Autodesk Fusion 360 part; units mm, degrees
note: some values were not read from the file. Chosen so that the rebuilt part matches the saved one: which face or edge a step refers to; which pieces of a blend or face edit are solid. Set by a fixed rule: which sketch regions a step uses.
(part 2 of 5)
  line L115 (-88.0068, -37.0951) -> (-84.7252, -33.8135)
  arc A155 (49.1749, 62.2927) -> (41.7643, 61.9168) centre (45.6394, 58.7571) ccw
  line L116 (38.5865, -65.8101) -> (15.8059, -43.0296)
  line L117 (-65.8101, -38.5865) -> (-43.0296, -15.8059)
  line L118 (-42.4797, -62.6322) -> (-23.3401, -43.4926)
  arc A156 (84.7263, -33.8146) -> (84.7252, -33.8135) centre (81.1896, -37.349) ccw
  line L119 (0, 0) -> (0, -10)
  arc A157 (84.7252, -33.8135) -> (77.6541, -33.8135) centre (81.1896, -37.349) ccw
  line L120 (33.8327, -77.6349) -> (33.8316, -77.636)
  line L121 (38.6227, -72.8449) -> (33.8139, -77.6537)
  arc A158 (-49.1749, -62.2927) -> (-41.7643, -61.9168) centre (-45.6394, -58.7571) ccw
  line L122 (77.653, -33.8146) -> (77.6541, -33.8135)
  line L123 (72.8449, -38.6227) -> (72.863, -38.6046)
  line L124 (-84.7081, -33.8327) -> (-84.707, -33.8316)
  line L125 (-38.6046, -72.863) -> (-72.8811, -38.5865)
  arc A159 (38.5865, -72.8811) -> (38.5865, -65.8101) centre (35.0509, -69.3456) ccw
  arc A160 (-72.8811, -38.5865) -> (-65.8101, -38.5865) centre (-69.3456, -35.0509) ccw
  line L126 (42.122, -62.2745) -> (23.3401, -43.4926)
  arc A161 (62.2745, 42.122) -> (62.2745, 49.1931) centre (58.739, 45.6575) ccw
  line L127 (62.6322, -42.4797) -> (43.4926, -23.3401)
  line L128 (-42.122, 62.2745) -> (-23.3401, 43.4926)
  arc A162 (-65.4524, 38.2288) -> (-72.863, 38.6046) centre (-69.3275, 35.0691) ccw
  line L129 (62.2745, 42.122) -> (43.4926, 23.3401)
  line L130 (-72.863, 38.6046) -> (-77.6541, 33.8135)
  arc A163 (65.4524, -38.2288) -> (72.863, -38.6046) centre (69.3275, -35.0691) ccw
  arc A164 (33.8139, -77.6537) -> (33.7586, -84.6686) centre (37.3495, -81.1892) ccw
  line L131 (-55.7429, 55.7247) -> (-52.8534, 52.8352)
  arc A165 (-62.2745, -42.122) -> (-62.2745, -49.1931) centre (-58.739, -45.6575) ccw
  line L132 (-38.5865, 65.8101) -> (-15.8059, 43.0296)
  arc A166 (-38.5865, 72.8811) -> (-38.5865, 65.8101) centre (-35.0509, 69.3456) ccw
  line L133 (66.1678, -38.9441) -> (43.0296, -15.8059)
  line L134 (72.8449, 38.6227) -> (77.636, 33.8316)
  line L135 (72.8449, -38.6227) -> (77.6541, -33.8135)
  line L136 (38.6227, -72.8449) -> (38.5865, -72.8811)
  line L137 (42.4797, 62.6322) -> (23.3401, 43.4926)
  line L138 (35.2277, -86.1394) -> (33.8135, -84.7252)
  line L139 (87.9887, 37.1133) -> (84.707, 33.8316)
  line L140 (-37.1133, 87.9887) -> (-33.8316, 84.707)
  arc A167 (42.122, -62.2745) -> (49.1931, -62.2745) centre (45.6575, -58.739) ccw
  line L141 (37.0951, 88.0068) -> (33.8135, 84.7252)
  line L142 (-62.2745, -42.122) -> (-43.4926, -23.3401)
  line L143 (-77.636, -33.8316) -> (-77.6541, -33.8135)
  arc A168 (-33.8327, 77.6349) -> (-33.8327, 84.7081) centre (-37.3672, 81.1715) ccw
  arc A169 (62.2927, -49.1749) -> (61.9168, -41.7643) centre (58.7571, -45.6394) ccw
  line L144 (38.6046, 72.863) -> (33.8135, 77.6541)
  line L145 (-38.6046, -72.863) -> (-33.8135, -77.6541)
  line L146 (33.8135, -84.7252) -> (33.7586, -84.6686)
  line L147 (72.863, -38.6046) -> (38.5865, -72.8811)
  line L148 (-66.1678, 38.9441) -> (-43.0296, 15.8059)
  arc A170 (-33.8146, -84.7263) -> (-33.8146, -77.653) centre (-37.349, -81.1896) ccw
  line L149 (-72.8449, -38.6227) -> (-77.636, -33.8316)
  line L150 (-37.0951, -88.0068) -> (-33.8135, -84.7252)
  arc A171 (-77.6541, -33.8135) -> (-84.7252, -33.8135) centre (-81.1896, -37.349) ccw
  point P0 (-86.1394, -35.2277)
  point P1 (35.2277, -86.1394)
  point P2 (86.1394, 35.2277)
  point P3 (86.1394, 35.2277)
  point P4 (-86.1394, -35.2277)
  point P5 (35.2277, -86.1394)
  dimension "d63" = 5
  dimension "d64" = 5
  dimension "d67" = 5
  dimension "d82" = 5
  dimension "d83" = 5
  dimension "d84" = 5
  constraint concentric A25 A123
  constraint concentric A76 A124
  constraint concentric A77 A125
  constraint concentric A81 A126
  constraint coincident A25.start L16.start
  constraint coincident L16.end A26.end
  constraint coincident L39.end A76.end
  constraint coincident L39.start A80.start
  constraint coincident A77.start L41.start
  constraint tangent L64 A125
  constraint parallel L41 L64
  constraint coincident A81.end L45.end
  constraint coincident A88.start L45.start
  constraint coincident L15.end A25.end
  constraint coincident A24.end L15.start
  constraint coincident A23.start L14.start
  constraint coincident L14.end A24.start
  constraint concentric A24 A122
  constraint coincident A24.end A122
  constraint coincident L14 A122.start
  constraint coincident L15 A122.end
  constraint coincident L16 A123.start
  constraint coincident L39 A124.end
  constraint midpoint L40 L68.start
  constraint perpendicular L40 L68
  constraint symmetric L15.end L68 L70.start
  constraint symmetric A24.end L68 L70.end
  constraint symmetric A23.start L68 L69.start
  constraint symmetric L14.end L68 L69.end
  constraint symmetric A122 L68 A127
  constraint symmetric A122.start L68 A127.end
  constraint symmetric A122.end L68 A127.start
  constraint coincident L13.end A21.end
  constraint tangent A21 L95
  constraint perpendicular L95 L96
  constraint tangent L96 A144
  constraint tangent L95 A144
  constraint coincident A5.centre A10.centre
  constraint vertical L97
  constraint symmetric L74.start L97 L98.start
  constraint coincident A63.start L29.start
  constraint tangent A63 L99
  constraint perpendicular L99 L100
  constraint tangent L99 A145
  constraint tangent L100 A145
  constraint collinear L101 L102
  constraint parallel L81 L103
  constraint coincident P5 P1
  constraint perpendicular L103 L104
  constraint parallel L3 L105
  constraint tangent L103 A146
  constraint tangent L105 A146
  constraint tangent A152 L128
  constraint coincident A24.end A151
  constraint symmetric L15.end L70.start L131
  constraint symmetric A24.end L70.end L131
  constraint symmetric A23.start L69.start L131
  constraint symmetric L14.end L69.end L131
  constraint symmetric A151 L131 A168
  constraint symmetric A122.start A127.end L131
  constraint symmetric A122.end A127.start L131
  constraint perpendicular L115 L143
  constraint tangent L143 A171
  constraint tangent L115 A171
  constraint vertical L119
  constraint symmetric L74.start L98.start L119
  constraint perpendicular L107 L135
  constraint tangent L107 A157
  constraint tangent A157 L135
  constraint collinear L120 L136
  constraint parallel L121 L147
  constraint perpendicular L121 L138
  constraint tangent L121 A164
  constraint tangent A164 L146
  measures "d63" radius of A144
  measures "d64" radius of A145
  measures "d67" radius of A146
  measures "d82" radius of A171
  measures "d83" radius of A157
  measures "d84" radius of A164
extrude "押し出し10" cut sketch "スケッチ2" against normal blind 100 contours L6 A12 L7 A13 A128 L72 A132 A148 L145 A170 | A14 L9 A15 L73 L77 A130 A131 A158 L125 A165 L142 | A19 L12 A20 L13 L73 L74 A129 L76 L96 A144 L117 L125 A160 L143 L149 A171 | A7 L2 A8 L3 L81 A134 L101 L103 A146 L121 A159 A164 L136 L147 | L36 L81 A135 A136 A167 A169 L147 | L29 A64 L30 A65 A133 L81 A137 L84 L98 L100 A145 A156 A157 L123 A163 L133 L135 L147 | A118 L53 L54 A119 L55 L56 A120 L57 L58 A121 L59 L60 bodies 1
extrude "押し出し11" add sketch "スケッチ2" against normal blind 1.5 contours L36 L37 L38 A135 A167 | L35 L36 A136 A169 bodies 1
sketch "スケッチ4" plane through (0, 0, 0) normal (0, 0, -1) x (1, 0, 0)
  arc A0 (17.125, 34.0956) -> (-17.125, 34.0956) centre (0, 0) ccw
  line L0 (17.125, 34.0956) -> (17.1965, 34.167)
  line L1 (17.1965, 34.167) -> (17.4152, 33.9483)
  arc A1 (33.9483, 17.4152) -> (17.4152, 33.9483) centre (0, 0) ccw
  line L2 (33.9483, 17.4152) -> (34.167, 17.1965)
  line L3 (34.167, 17.1965) -> (34.0956, 17.125)
  arc A2 (-34.0956, 17.125) -> (34.0956, 17.125) centre (0, 0) ccw
  line L4 (-34.0956, 17.125) -> (-34.167, 17.1965)
  line L5 (-34.167, 17.1965) -> (-33.9483, 17.4152)
  arc A3 (-17.4152, 33.9483) -> (-33.9483, 17.4152) centre (0, 0) ccw
  line L6 (-17.4152, 33.9483) -> (-17.1965, 34.167)
  line L7 (-17.1965, 34.167) -> (-17.125, 34.0956)
  circle A4 centre (-39.2089, -15.5208) radius 1.75
  circle A5 centre (-15.5208, -39.2089) radius 1.75
  circle A6 centre (-26.1275, -49.8155) radius 1.75
  circle A7 centre (-49.8155, -26.1275) radius 1.75
  arc A8 (32.3993, 86.1394) -> (35.2277, 86.1394) centre (33.8135, 87.5536) ccw
  line L8 (32.3993, 86.1394) -> (26.1835, 92.3551)
  arc A9 (25.9652, 94.9247) -> (26.1835, 92.3551) centre (27.5978, 93.7693) ccw
  arc A10 (25.9652, 94.9247) -> (26.3162, 95.431) centre (0, 113.3) ccw
  arc A11 (32.0144, 97.3721) -> (26.3162, 95.431) centre (30.4528, 92.6222) ccw
  arc A12 (39.6929, 94.5025) -> (32.0144, 97.3721) centre (0, 0) ccw
  arc A13 (40.3326, 91.2443) -> (39.6929, 94.5025) centre (38.9184, 92.6585) ccw
  line L9 (40.3326, 91.2443) -> (35.2277, 86.1394)
  circle A14 centre (26.1275, 49.8155) radius 1.75
  arc A15 (23.3401, 43.4926) -> (24.0851, 35.8083) centre (26.8756, 39.9571) ccw
  line L10 (23.3401, 43.4926) -> (42.122, 62.2745)
  arc A16 (49.1931, 62.2745) -> (42.122, 62.2745) centre (45.6575, 58.739) ccw
  line L11 (49.1931, 62.2745) -> (62.2927, 49.1749)
  arc A17 (62.6322, 42.4797) -> (62.2927, 49.1749) centre (58.7571, 45.6394) ccw
  line L12 (62.6322, 42.4797) -> (43.4926, 23.3401)
  arc A18 (35.8083, 24.0851) -> (43.4926, 23.3401) centre (39.9571, 26.8756) ccw
  arc A19 (35.8083, 24.0851) -> (24.0851, 35.8083) centre (0, 0) ccw
  circle A20 centre (49.8155, -26.1275) radius 1.75
  circle A21 centre (49.8155, 26.1275) radius 1.75
  circle A22 centre (15.5208, 39.2089) radius 1.75
  circle A23 centre (26.1275, -49.8155) radius 1.75
  circle A24 centre (39.2089, 15.5208) radius 1.75
  circle A25 centre (15.5208, -39.2089) radius 1.75
  circle A26 centre (39.2089, -15.5208) radius 1.75
  line L13 (-35.2277, 86.1394) -> (-40.3326, 91.2443)
  arc A27 (-39.6929, 94.5025) -> (-40.3326, 91.2443) centre (-38.9184, 92.6585) ccw
  arc A28 (-32.0144, 97.3721) -> (-39.6929, 94.5025) centre (0, 0) ccw
  arc A29 (-26.3162, 95.431) -> (-32.0144, 97.3721) centre (-30.4528, 92.6222) ccw
  arc A30 (-26.3162, 95.431) -> (-25.9652, 94.9247) centre (0, 113.3) ccw
  arc A31 (-26.1835, 92.3551) -> (-25.9652, 94.9247) centre (-27.5978, 93.7693) ccw
  line L14 (-26.1835, 92.3551) -> (-32.3993, 86.1394)
  arc A32 (-35.2277, 86.1394) -> (-32.3993, 86.1394) centre (-33.8135, 87.5536) ccw
  arc A33 (-38.5865, 72.8811) -> (-38.5865, 65.8101) centre (-35.0509, 69.3456) ccw
  line L15 (-38.5865, 72.8811) -> (-24.7285, 86.7391)
  arc A34 (-18.3143, 87.2917) -> (-24.7285, 86.7391) centre (-21.193, 83.2035) ccw
  arc A35 (-18.3143, 87.2917) -> (18.3143, 87.2917) centre (0, 113.3) ccw
  arc A36 (24.7285, 86.7391) -> (18.3143, 87.2917) centre (21.193, 83.2035) ccw
  line L16 (24.7285, 86.7391) -> (38.5865, 72.8811)
  arc A37 (38.5865, 65.8101) -> (38.5865, 72.8811) centre (35.0509, 69.3456) ccw
  line L17 (38.5865, 65.8101) -> (15.8059, 43.0296)
  arc A38 (10.9963, 41.7301) -> (15.8059, 43.0296) centre (12.2704, 46.5651) ccw
  arc A39 (10.9963, 41.7301) -> (-10.9963, 41.7301) centre (0, 0) ccw
  arc A40 (-15.8059, 43.0296) -> (-10.9963, 41.7301) centre (-12.2704, 46.5651) ccw
  line L18 (-15.8059, 43.0296) -> (-38.5865, 65.8101)
  line L19 (-43.4926, 23.3401) -> (-62.6322, 42.4797)
  arc A41 (-62.2927, 49.1749) -> (-62.6322, 42.4797) centre (-58.7571, 45.6394) ccw
  line L20 (-62.2927, 49.1749) -> (-49.1931, 62.2745)
  arc A42 (-42.122, 62.2745) -> (-49.1931, 62.2745) centre (-45.6575, 58.739) ccw
  line L21 (-42.122, 62.2745) -> (-23.3401, 43.4926)
  arc A43 (-24.0851, 35.8083) -> (-23.3401, 43.4926) centre (-26.8756, 39.9571) ccw
  arc A44 (-24.0851, 35.8083) -> (-35.8083, 24.0851) centre (0, 0) ccw
  arc A45 (-43.4926, 23.3401) -> (-35.8083, 24.0851) centre (-39.9571, 26.8756) ccw
  arc A46 (62.2927, -49.1749) -> (62.6322, -42.4797) centre (58.7571, -45.6394) ccw
  line L22 (62.2927, -49.1749) -> (49.1931, -62.2745)
  arc A47 (42.122, -62.2745) -> (49.1931, -62.2745) centre (45.6575, -58.739) ccw
  line L23 (42.122, -62.2745) -> (23.3401, -43.4926)
  arc A48 (24.0851, -35.8083) -> (23.3401, -43.4926) centre (26.8756, -39.9571) ccw
  arc A49 (24.0851, -35.8083) -> (35.8083, -24.0851) centre (0, 0) ccw
  arc A50 (43.4926, -23.3401) -> (35.8083, -24.0851) centre (39.9571, -26.8756) ccw
  line L24 (43.4926, -23.3401) -> (62.6322, -42.4797)
  arc A51 (84.7252, -33.8135) -> (77.6541, -33.8135) centre (81.1896, -37.349) ccw
  line L25 (77.6541, -33.8135) -> (72.863, -38.6046)
  arc A52 (66.1678, -38.9441) -> (72.863, -38.6046) centre (69.3275, -35.0691) ccw
  line L26 (66.1678, -38.9441) -> (63.9577, -36.7341)
  line L27 (63.9577, -36.7341) -> (43.0296, -15.8059)
  arc A53 (41.7301, -10.9963) -> (43.0296, -15.8059) centre (46.5651, -12.2704) ccw
  arc A54 (41.7301, -10.9963) -> (41.7301, 10.9963) centre (0, 0) ccw
  arc A55 (43.0296, 15.8059) -> (41.7301, 10.9963) centre (46.5651, 12.2704) ccw
  line L28 (43.0296, 15.8059) -> (66.1678, 38.9441)
  arc A56 (72.863, 38.6046) -> (66.1678, 38.9441) centre (69.3275, 35.0691) ccw
  line L29 (72.863, 38.6046) -> (77.6541, 33.8135)
  arc A57 (77.6541, 33.8135) -> (84.7252, 33.8135) centre (81.1896, 37.349) ccw
  line L30 (84.7252, 33.8135) -> (88.0068, 37.0951)
  arc A58 (96.2368, 35.2806) -> (88.0068, 37.0951) centre (91.5424, 33.5596) ccw
  arc A59 (96.2368, -35.2806) -> (96.2368, 35.2806) centre (0, 0) ccw
  arc A60 (88.0068, -37.0951) -> (96.2368, -35.2806) centre (91.5424, -33.5596) ccw
  line L31 (88.0068, -37.0951) -> (84.7252, -33.8135)
  arc A61 (-90.783, -46.7156) -> (-91.4938, -47.061) centre (-91.0045, -47.1639) ccw
  arc A62 (-90.783, -46.7156) -> (-89.7814, -45.9408) centre (-93.3169, -42.4052) ccw
  line L32 (-89.7814, -45.9408) -> (-84.7252, -40.8846)
  arc A63 (-77.6541, -40.8846) -> (-84.7252, -40.8846) centre (-81.1896, -44.4201) ccw
  line L33 (-77.6541, -40.8846) -> (-40.8846, -77.6541)
  arc A64 (-40.8846, -84.7252) -> (-40.8846, -77.6541) centre (-44.4201, -81.1896) ccw
  line L34 (-40.8846, -84.7252) -> (-45.9408, -89.7814)
  arc A65 (-45.9408, -89.7814) -> (-44.4738, -97.869) centre (-42.4052, -93.3169) ccw
  arc A66 (-44.4738, -97.869) -> (44.4738, -97.869) centre (0, 0) ccw
  arc A67 (44.4738, -97.869) -> (45.9408, -89.7814) centre (42.4052, -93.3169) ccw
  line L35 (45.9408, -89.7814) -> (40.8846, -84.7252)
  arc A68 (40.8846, -77.6541) -> (40.8846, -84.7252) centre (44.4201, -81.1896) ccw
  line L36 (40.8846, -77.6541) -> (77.6541, -40.8846)
  arc A69 (84.7252, -40.8846) -> (77.6541, -40.8846) centre (81.1896, -44.4201) ccw
  line L37 (84.7252, -40.8846) -> (89.7814, -45.9408)
  arc A70 (89.7814, -45.9408) -> (90.783, -46.7156) centre (93.3169, -42.4052) ccw
  arc A71 (91.4938, -47.061) -> (90.783, -46.7156) centre (91.0045, -47.1639) ccw
  arc A72 (91.4938, -47.061) -> (97.869, -44.4738) centre (93.3169, -42.4052) ccw
  arc A73 (97.869, -44.4738) -> (97.869, 44.4738) centre (0, 0) ccw
  arc A74 (97.869, 44.4738) -> (89.7814, 45.9408) centre (93.3169, 42.4052) ccw
  line L38 (89.7814, 45.9408) -> (84.7252, 40.8846)
  arc A75 (77.6541, 40.8846) -> (84.7252, 40.8846) centre (81.1896, 44.4201) ccw
  line L39 (77.6541, 40.8846) -> (40.8846, 77.6541)
  arc A76 (40.8846, 84.7252) -> (40.8846, 77.6541) centre (44.4201, 81.1896) ccw
  line L40 (40.8846, 84.7252) -> (45.9408, 89.7814)
  arc A77 (45.9408, 89.7814) -> (44.4738, 97.869) centre (42.4052, 93.3169) ccw
  arc A78 (44.4738, 97.869) -> (37.9262, 100.5876) centre (0, 0) ccw
  arc A79 (37.9256, 100.5859) -> (37.9262, 100.5876) centre (0, 113.3) ccw
  arc A80 (37.9256, 100.5859) -> (37.8014, 100.6345) centre (36.0432, 95.9538) ccw
  arc A81 (37.8014, 100.6345) -> (29.5575, 103.3567) centre (0, 0) ccw
  arc A82 (29.5575, 103.3567) -> (23.7528, 100.868) centre (28.1827, 98.5494) ccw
  arc A83 (-23.7528, 100.868) -> (23.7528, 100.868) centre (0, 113.3) ccw
  arc A84 (-23.7528, 100.868) -> (-29.5575, 103.3567) centre (-28.1827, 98.5494) ccw
  arc A85 (-29.5575, 103.3567) -> (-37.8014, 100.6345) centre (0, 0) ccw
  arc A86 (-37.8014, 100.6345) -> (-37.9256, 100.5859) centre (-36.0432, 95.9538) ccw
  arc A87 (-37.9262, 100.5876) -> (-37.9256, 100.5859) centre (0, 113.3) ccw
  arc A88 (-37.9262, 100.5876) -> (-44.4738, 97.869) centre (0, 0) ccw
  arc A89 (-44.4738, 97.869) -> (-45.9408, 89.7814) centre (-42.4052, 93.3169) ccw
  line L41 (-45.9408, 89.7814) -> (-40.8846, 84.7252)
  arc A90 (-40.8846, 77.6541) -> (-40.8846, 84.7252) centre (-44.4201, 81.1896) ccw
  line L42 (-40.8846, 77.6541) -> (-77.6541, 40.8846)
  arc A91 (-84.7252, 40.8846) -> (-77.6541, 40.8846) centre (-81.1896, 44.4201) ccw
  line L43 (-84.7252, 40.8846) -> (-89.7814, 45.9408)
  arc A92 (-89.7814, 45.9408) -> (-97.869, 44.4738) centre (-93.3169, 42.4052) ccw
  arc A93 (-97.869, 44.4738) -> (-97.869, -44.4738) centre (0, 0) ccw
  arc A94 (-97.869, -44.4738) -> (-91.4938, -47.061) centre (-93.3169, -42.4052) ccw
  line L44 (-63.9577, -36.7341) -> (-65.8101, -38.5865)
  arc A95 (-72.8811, -38.5865) -> (-65.8101, -38.5865) centre (-69.3456, -35.0509) ccw
  line L45 (-72.8811, -38.5865) -> (-77.6541, -33.8135)
  arc A96 (-77.6541, -33.8135) -> (-84.7252, -33.8135) centre (-81.1896, -37.349) ccw
  line L46 (-84.7252, -33.8135) -> (-88.0068, -37.0951)
  arc A97 (-96.2368, -35.2806) -> (-88.0068, -37.0951) centre (-91.5424, -33.5596) ccw
  arc A98 (-96.2368, 35.2806) -> (-96.2368, -35.2806) centre (0, 0) ccw
  arc A99 (-88.0068, 37.0951) -> (-96.2368, 35.2806) centre (-91.5424, 33.5596) ccw
  line L47 (-88.0068, 37.0951) -> (-84.7252, 33.8135)
  arc A100 (-84.7252, 33.8135) -> (-77.6541, 33.8135) centre (-81.1896, 37.349) ccw
  line L48 (-77.6541, 33.8135) -> (-72.863, 38.6046)
  arc A101 (-66.1678, 38.9441) -> (-72.863, 38.6046) centre (-69.3275, 35.0691) ccw
  line L49 (-66.1678, 38.9441) -> (-43.0296, 15.8059)
  arc A102 (-41.7301, 10.9963) -> (-43.0296, 15.8059) centre (-46.5651, 12.2704) ccw
  arc A103 (-41.7301, 10.9963) -> (-41.7301, -10.9963) centre (0, 0) ccw
  arc A104 (-43.0296, -15.8059) -> (-41.7301, -10.9963) centre (-46.5651, -12.2704) ccw
  line L50 (-43.0296, -15.8059) -> (-63.9577, -36.7341)
  arc A105 (-49.1749, -62.2927) -> (-42.4797, -62.6322) centre (-45.6394, -58.7571) ccw
  line L51 (-49.1749, -62.2927) -> (-62.2745, -49.1931)
  arc A106 (-62.2745, -42.122) -> (-62.2745, -49.1931) centre (-58.739, -45.6575) ccw
  line L52 (-62.2745, -42.122) -> (-43.4926, -23.3401)
  arc A107 (-35.8083, -24.0851) -> (-43.4926, -23.3401) centre (-39.9571, -26.8756) ccw
  arc A108 (-35.8083, -24.0851) -> (-24.0851, -35.8083) centre (0, 0) ccw
  arc A109 (-23.3401, -43.4926) -> (-24.0851, -35.8083) centre (-26.8756, -39.9571) ccw
  line L53 (-23.3401, -43.4926) -> (-42.4797, -62.6322)
  arc A110 (-33.7038, -84.612) -> (-33.8146, -77.653) centre (-37.349, -81.1896) ccw
  line L54 (-33.8146, -77.653) -> (-38.6046, -72.863)
  arc A111 (-38.9441, -66.1678) -> (-38.6046, -72.863) centre (-35.0691, -69.3275) ccw
  line L55 (-38.9441, -66.1678) -> (-15.8059, -43.0296)
  arc A112 (-10.9963, -41.7301) -> (-15.8059, -43.0296) centre (-12.2704, -46.5651) ccw
  arc A113 (-10.9963, -41.7301) -> (10.9963, -41.7301) centre (0, 0) ccw
  arc A114 (15.8059, -43.0296) -> (10.9963, -41.7301) centre (12.2704, -46.5651) ccw
  line L56 (15.8059, -43.0296) -> (38.9441, -66.1678)
  arc A115 (38.9491, -66.2144) -> (38.9441, -66.1678) centre (33.9744, -66.7173) ccw
  arc A116 (38.5865, -72.8811) -> (38.9491, -66.2144) centre (35.0509, -69.3456) ccw
  line L57 (38.5865, -72.8811) -> (33.8139, -77.6537)
  arc A117 (33.8139, -77.6537) -> (33.7586, -84.6686) centre (37.3495, -81.1892) ccw
  line L58 (33.7586, -84.6686) -> (33.8135, -84.7252)
  line L59 (33.8135, -84.7252) -> (37.0951, -88.0068)
  arc A118 (35.2806, -96.2368) -> (37.0951, -88.0068) centre (33.5596, -91.5424) ccw
  arc A119 (-35.2806, -96.2368) -> (35.2806, -96.2368) centre (0, 0) ccw
  arc A120 (-37.0951, -88.0068) -> (-35.2806, -96.2368) centre (-33.5596, -91.5424) ccw
  line L60 (-37.0951, -88.0068) -> (-33.8135, -84.7252)
  line L61 (-33.8135, -84.7252) -> (-33.7038, -84.612)
  circle A121 centre (-49.8155, 26.1275) radius 1.75
  circle A122 centre (-15.5208, 39.2089) radius 1.75
  circle A123 centre (-39.2089, 15.5208) radius 1.75
  circle A124 centre (-26.1275, 49.8155) radius 1.75
  circle A125 centre (-32.1379, -59.3615) radius 1.75
  circle A126 centre (32.1379, -59.3615) radius 1.75
  circle A127 centre (-32.1379, -59.3615) radius 2.5
  circle A128 centre (32.1379, -59.3615) radius 2.5
  dimension "d89" = 3.5
  dimension "d90" = 3.5
  dimension "d91" = 5
  dimension "d92" = 5
  constraint concentric A125 A127
  constraint concentric A126 A128
  measures "d89" diameter of A125
  measures "d90" diameter of A126
  measures "d91" diameter of A127
  measures "d92" diameter of A128
extrude "押し出し12" add sketch "スケッチ4" against normal blind 1.5 contours L55 A125 A127 | L55 A125 A127 | L56 A126 A128 picked at (33.5684, -61.0906) bodies 1
extrude "押し出し13" cut sketch "スケッチ4" against normal blind 1.5 contours L55 A125 | L55 A125 | L56 A126 picked at (32.0241, -58.7893) bodies 1
fillet "フィレット4" radius 5 4 edges at (-30.3701, 57.5937, 0.75) (-33.9056, 61.1292, 0.75) (33.9056, 61.1292, 0.75) (30.3701, 57.5937, 0.75) on bodies 1
sketch "スケッチ5" plane through (0, 0, 1.5) normal (0, 0, 1) x (-1, 0, 0)
  circle A0 centre (39.2089, -15.5208) radius 1.75
  circle A1 centre (15.5208, -39.2089) radius 1.75
  circle A2 centre (26.1275, -49.8155) radius 1.75
  circle A3 centre (49.8155, -26.1275) radius 1.75
  arc A4 (-35.2277, 86.1394) -> (-32.3993, 86.1394) centre (-33.8135, 87.5536) ccw
  line L0 (-35.2277, 86.1394) -> (-40.3326, 91.2443)
  arc A5 (-39.6929, 94.5025) -> (-40.3326, 91.2443) centre (-38.9184, 92.6585) ccw
  arc A6 (-32.0144, 97.3721) -> (-39.6929, 94.5025) centre (0, 0) ccw
  arc A7 (-26.3162, 95.431) -> (-32.0144, 97.3721) centre (-30.4528, 92.6222) ccw
  arc A8 (-26.3162, 95.431) -> (-25.9652, 94.9247) centre (0, 113.3) ccw
  arc A9 (-26.1835, 92.3551) -> (-25.9652, 94.9247) centre (-27.5978, 93.7693) ccw
  line L1 (-26.1835, 92.3551) -> (-32.3993, 86.1394)
  circle A10 centre (-26.1275, 49.8155) radius 1.75
  arc A11 (-24.0851, 35.8083) -> (-23.3401, 43.4926) centre (-26.8756, 39.9571) ccw
  arc A12 (-24.0851, 35.8083) -> (-35.8083, 24.0851) centre (0, 0) ccw
  arc A13 (-43.4926, 23.3401) -> (-35.8083, 24.0851) centre (-39.9571, 26.8756) ccw
  line L2 (-43.4926, 23.3401) -> (-62.6322, 42.4797)
  arc A14 (-62.2927, 49.1749) -> (-62.6322, 42.4797) centre (-58.7571, 45.6394) ccw
  line L3 (-62.2927, 49.1749) -> (-49.1931, 62.2745)
  arc A15 (-42.122, 62.2745) -> (-49.1931, 62.2745) centre (-45.6575, 58.739) ccw
  line L4 (-42.122, 62.2745) -> (-23.3401, 43.4926)
  circle A16 centre (-49.8155, -26.1275) radius 1.75
  circle A17 centre (-49.8155, 26.1275) radius 1.75
  circle A18 centre (-15.5208, 39.2089) radius 1.75
  circle A19 centre (-26.1275, -49.8155) radius 1.75
  circle A20 centre (-39.2089, 15.5208) radius 1.75
  circle A21 centre (-15.5208, -39.2089) radius 1.75
  circle A22 centre (-39.2089, -15.5208) radius 1.75
  line L5 (40.3326, 91.2443) -> (35.2277, 86.1394)
  arc A23 (32.3993, 86.1394) -> (35.2277, 86.1394) centre (33.8135, 87.5536) ccw
  line L6 (32.3993, 86.1394) -> (26.1835, 92.3551)
  arc A24 (25.9652, 94.9247) -> (26.1835, 92.3551) centre (27.5978, 93.7693) ccw
  arc A25 (25.9652, 94.9247) -> (26.3162, 95.431) centre (0, 113.3) ccw
  arc A26 (32.0144, 97.3721) -> (26.3162, 95.431) centre (30.4528, 92.6222) ccw
  arc A27 (39.6929, 94.5025) -> (32.0144, 97.3721) centre (0, 0) ccw
  arc A28 (40.3326, 91.2443) -> (39.6929, 94.5025) centre (38.9184, 92.6585) ccw
  arc A29 (17.125, 34.0956) -> (-17.125, 34.0956) centre (0, 0) ccw
  line L7 (17.125, 34.0956) -> (17.1965, 34.167)
  line L8 (17.1965, 34.167) -> (17.4152, 33.9483)
  arc A30 (33.9483, 17.4152) -> (17.4152, 33.9483) centre (0, 0) ccw
  line L9 (33.9483, 17.4152) -> (34.167, 17.1965)
  line L10 (34.167, 17.1965) -> (34.0956, 17.125)
  arc A31 (-34.0956, 17.125) -> (34.0956, 17.125) centre (0, 0) ccw
  line L11 (-34.0956, 17.125) -> (-34.167, 17.1965)
  line L12 (-34.167, 17.1965) -> (-33.9483, 17.4152)
  arc A32 (-17.4152, 33.9483) -> (-33.9483, 17.4152) centre (0, 0) ccw
  line L13 (-17.4152, 33.9483) -> (-17.1965, 34.167)
  line L14 (-17.1965, 34.167) -> (-17.125, 34.0956)
  line L15 (38.5865, 65.8101) -> (15.8059, 43.0296)
  arc A33 (10.9963, 41.7301) -> (15.8059, 43.0296) centre (12.2704, 46.5651) ccw
  arc A34 (10.9963, 41.7301) -> (-10.9963, 41.7301) centre (0, 0) ccw
  arc A35 (-15.8059, 43.0296) -> (-10.9963, 41.7301) centre (-12.2704, 46.5651) ccw
  line L16 (-15.8059, 43.0296) -> (-38.5865, 65.8101)
  arc A36 (-38.5865, 72.8811) -> (-38.5865, 65.8101) centre (-35.0509, 69.3456) ccw
  line L17 (-38.5865, 72.8811) -> (-24.7285, 86.7391)
  arc A37 (-18.3143, 87.2917) -> (-24.7285, 86.7391) centre (-21.193, 83.2035) ccw
  arc A38 (-18.3143, 87.2917) -> (18.3143, 87.2917) centre (0, 113.3) ccw
  arc A39 (24.7285, 86.7391) -> (18.3143, 87.2917) centre (21.193, 83.2035) ccw
  line L18 (24.7285, 86.7391) -> (38.5865, 72.8811)
  arc A40 (38.5865, 65.8101) -> (38.5865, 72.8811) centre (35.0509, 69.3456) ccw
  line L19 (62.6322, 42.4797) -> (43.4926, 23.3401)
  arc A41 (35.8083, 24.0851) -> (43.4926, 23.3401) centre (39.9571, 26.8756) ccw
  arc A42 (35.8083, 24.0851) -> (24.0851, 35.8083) centre (0, 0) ccw
  arc A43 (23.3401, 43.4926) -> (24.0851, 35.8083) centre (26.8756, 39.9571) ccw
  line L20 (23.3401, 43.4926) -> (42.122, 62.2745)
  arc A44 (49.1931, 62.2745) -> (42.122, 62.2745) centre (45.6575, 58.739) ccw
  line L21 (49.1931, 62.2745) -> (62.2927, 49.1749)
  arc A45 (62.6322, 42.4797) -> (62.2927, 49.1749) centre (58.7571, 45.6394) ccw
  arc A46 (91.4938, -47.061) -> (90.783, -46.7156) centre (91.0045, -47.1639) ccw
  arc A47 (91.4938, -47.061) -> (97.869, -44.4738) centre (93.3169, -42.4052) ccw
  arc A48 (97.869, -44.4738) -> (97.869, 44.4738) centre (0, 0) ccw
  arc A49 (97.869, 44.4738) -> (89.7814, 45.9408) centre (93.3169, 42.4052) ccw
  line L22 (89.7814, 45.9408) -> (84.7252, 40.8846)
  arc A50 (77.6541, 40.8846) -> (84.7252, 40.8846) centre (81.1896, 44.4201) ccw
  line L23 (77.6541, 40.8846) -> (40.8846, 77.6541)
  arc A51 (40.8846, 84.7252) -> (40.8846, 77.6541) centre (44.4201, 81.1896) ccw
  line L24 (40.8846, 84.7252) -> (45.9408, 89.7814)
  arc A52 (45.9408, 89.7814) -> (44.4738, 97.869) centre (42.4052, 93.3169) ccw
  arc A53 (44.4738, 97.869) -> (37.9262, 100.5876) centre (0, 0) ccw
  arc A54 (37.9256, 100.5859) -> (37.9262, 100.5876) centre (0, 113.3) ccw
  arc A55 (37.9256, 100.5859) -> (37.8014, 100.6345) centre (36.0432, 95.9538) ccw
  arc A56 (37.8014, 100.6345) -> (29.5575, 103.3567) centre (0, 0) ccw
  arc A57 (29.5575, 103.3567) -> (23.7528, 100.868) centre (28.1827, 98.5494) ccw
  arc A58 (-23.7528, 100.868) -> (23.7528, 100.868) centre (0, 113.3) ccw
  arc A59 (-23.7528, 100.868) -> (-29.5575, 103.3567) centre (-28.1827, 98.5494) ccw
  arc A60 (-29.5575, 103.3567) -> (-37.8014, 100.6345) centre (0, 0) ccw
  arc A61 (-37.8014, 100.6345) -> (-37.9256, 100.5859) centre (-36.0432, 95.9538) ccw
  arc A62 (-37.9262, 100.5876) -> (-37.9256, 100.5859) centre (0, 113.3) ccw
  arc A63 (-37.9262, 100.5876) -> (-44.4738, 97.869) centre (0, 0) ccw
  arc A64 (-44.4738, 97.869) -> (-45.9408, 89.7814) centre (-42.4052, 93.3169) ccw
  line L25 (-45.9408, 89.7814) -> (-40.8846, 84.7252)
  arc A65 (-40.8846, 77.6541) -> (-40.8846, 84.7252) centre (-44.4201, 81.1896) ccw
  line L26 (-40.8846, 77.6541) -> (-77.6541, 40.8846)
  arc A66 (-84.7252, 40.8846) -> (-77.6541, 40.8846) centre (-81.1896, 44.4201) ccw
  line L27 (-84.7252, 40.8846) -> (-89.7814, 45.9408)
  arc A67 (-89.7814, 45.9408) -> (-97.869, 44.4738) centre (-93.3169, 42.4052) ccw
  arc A68 (-97.869, 44.4738) -> (-97.869, -44.4738) centre (0, 0) ccw
  arc A69 (-97.869, -44.4738) -> (-91.4938, -47.061) centre (-93.3169, -42.4052) ccw
  arc A70 (-90.783, -46.7156) -> (-91.4938, -47.061) centre (-91.0045, -47.1639) ccw
  arc A71 (-90.783, -46.7156) -> (-89.7814, -45.9408) centre (-93.3169, -42.4052) ccw
  line L28 (-89.7814, -45.9408) -> (-84.7252, -40.8846)
  arc A72 (-77.6541, -40.8846) -> (-84.7252, -40.8846) centre (-81.1896, -44.4201) ccw
  line L29 (-77.6541, -40.8846) -> (-40.8846, -77.6541)
  arc A73 (-40.8846, -84.7252) -> (-40.8846, -77.6541) centre (-44.4201, -81.1896) ccw
  line L30 (-40.8846, -84.7252) -> (-45.9408, -89.7814)
  arc A74 (-45.9408, -89.7814) -> (-44.4738, -97.869) centre (-42.4052, -93.3169) ccw
  arc A75 (-44.4738, -97.869) -> (44.4738, -97.869) centre (0, 0) ccw
  arc A76 (44.4738, -97.869) -> (45.9408, -89.7814) centre (42.4052, -93.3169) ccw
  line L31 (45.9408, -89.7814) -> (40.8846, -84.7252)
  arc A77 (40.8846, -77.6541) -> (40.8846, -84.7252) centre (44.4201, -81.1896) ccw
  line L32 (40.8846, -77.6541) -> (77.6541, -40.8846)
  arc A78 (84.7252, -40.8846) -> (77.6541, -40.8846) centre (81.1896, -44.4201) ccw
  line L33 (84.7252, -40.8846) -> (89.7814, -45.9408)
  arc A79 (89.7814, -45.9408) -> (90.783, -46.7156) centre (93.3169, -42.4052) ccw
  circle A80 centre (49.8155, 26.1275) radius 1.75
  circle A81 centre (15.5208, 39.2089) radius 1.75
  circle A82 centre (39.2089, 15.5208) radius 1.75
  circle A83 centre (26.1275, 49.8155) radius 1.75
  line L34 (65.8101, -38.5865) -> (63.9577, -36.7341)
  line L35 (63.9577, -36.7341) -> (43.0296, -15.8059)
  arc A84 (41.7301, -10.9963) -> (43.0296, -15.8059) centre (46.5651, -12.2704) ccw
  arc A85 (41.7301, -10.9963) -> (41.7301, 10.9963) centre (0, 0) ccw
  arc A86 (43.0296, 15.8059) -> (41.7301, 10.9963) centre (46.5651, 12.2704) ccw
  line L36 (43.0296, 15.8059) -> (66.1678, 38.9441)
  arc A87 (72.863, 38.6046) -> (66.1678, 38.9441) centre (69.3275, 35.0691) ccw
  line L37 (72.863, 38.6046) -> (77.6541, 33.8135)
  arc A88 (77.6541, 33.8135) -> (84.7252, 33.8135) centre (81.1896, 37.349) ccw
  line L38 (84.7252, 33.8135) -> (88.0068, 37.0951)
  arc A89 (96.2368, 35.2806) -> (88.0068, 37.0951) centre (91.5424, 33.5596) ccw
  arc A90 (96.2368, -35.2806) -> (96.2368, 35.2806) centre (0, 0) ccw
  arc A91 (88.0068, -37.0951) -> (96.2368, -35.2806) centre (91.5424, -33.5596) ccw
  line L39 (88.0068, -37.0951) -> (84.7252, -33.8135)
  arc A92 (84.7252, -33.8135) -> (77.6541, -33.8135) centre (81.1896, -37.349) ccw
  line L40 (77.6541, -33.8135) -> (72.8811, -38.5865)
  arc A93 (65.8101, -38.5865) -> (72.8811, -38.5865) centre (69.3456, -35.0509) ccw
  arc A94 (42.4797, -62.6322) -> (49.1749, -62.2927) centre (45.6394, -58.7571) ccw
  line L41 (42.4797, -62.6322) -> (23.3401, -43.4926)
  arc A95 (24.0851, -35.8083) -> (23.3401, -43.4926) centre (26.8756, -39.9571) ccw
  arc A96 (24.0851, -35.8083) -> (35.8083, -24.0851) centre (0, 0) ccw
  arc A97 (43.4926, -23.3401) -> (35.8083, -24.0851) centre (39.9571, -26.8756) ccw
  line L42 (43.4926, -23.3401) -> (62.2745, -42.122)
  arc A98 (62.2745, -49.1931) -> (62.2745, -42.122) centre (58.739, -45.6575) ccw
  line L43 (62.2745, -49.1931) -> (49.1749, -62.2927)
  arc A99 (-77.6541, -33.8135) -> (-84.7252, -33.8135) centre (-81.1896, -37.349) ccw
  line L44 (-84.7252, -33.8135) -> (-88.0068, -37.0951)
  arc A100 (-96.2368, -35.2806) -> (-88.0068, -37.0951) centre (-91.5424, -33.5596) ccw
  arc A101 (-96.2368, 35.2806) -> (-96.2368, -35.2806) centre (0, 0) ccw
  arc A102 (-88.0068, 37.0951) -> (-96.2368, 35.2806) centre (-91.5424, 33.5596) ccw
  line L45 (-88.0068, 37.0951) -> (-84.7252, 33.8135)
  arc A103 (-84.7252, 33.8135) -> (-77.6541, 33.8135) centre (-81.1896, 37.349) ccw
  line L46 (-77.6541, 33.8135) -> (-72.863, 38.6046)
  arc A104 (-66.1678, 38.9441) -> (-72.863, 38.6046) centre (-69.3275, 35.0691) ccw
  line L47 (-66.1678, 38.9441) -> (-43.0296, 15.8059)
  arc A105 (-41.7301, 10.9963) -> (-43.0296, 15.8059) centre (-46.5651, 12.2704) ccw
  arc A106 (-41.7301, 10.9963) -> (-41.7301, -10.9963) centre (0, 0) ccw
  arc A107 (-43.0296, -15.8059) -> (-41.7301, -10.9963) centre (-46.5651, -12.2704) ccw
  line L48 (-43.0296, -15.8059) -> (-63.9577, -36.7341)
  line L49 (-63.9577, -36.7341) -> (-66.1678, -38.9441)
  arc A108 (-72.863, -38.6046) -> (-66.1678, -38.9441) centre (-69.3275, -35.0691) ccw
  line L50 (-72.863, -38.6046) -> (-77.6541, -33.8135)
  arc A109 (29.6417, -59.2224) -> (32.277, -61.8576) centre (32.1379, -59.3615) ccw
  arc A110 (36.0907, -63.3143) -> (32.277, -61.8576) centre (32.5552, -66.8499) ccw
  line L51 (36.0907, -63.3143) -> (38.9441, -66.1678)
  arc A111 (38.6046, -72.863) -> (38.9441, -66.1678) centre (35.0691, -69.3275) ccw
  line L52 (38.6046, -72.863) -> (33.8146, -77.653)
  arc A112 (33.8146, -77.653) -> (33.7038, -84.612) centre (37.349, -81.1896) ccw
  line L53 (33.7038, -84.612) -> (33.8135, -84.7252)
  line L54 (33.8135, -84.7252) -> (37.0951, -88.0068)
  arc A113 (35.2806, -96.2368) -> (37.0951, -88.0068) centre (33.5596, -91.5424) ccw
  arc A114 (-35.2806, -96.2368) -> (35.2806, -96.2368) centre (0, 0) ccw
  arc A115 (-37.0951, -88.0068) -> (-35.2806, -96.2368) centre (-33.5596, -91.5424) ccw
  line L55 (-37.0951, -88.0068) -> (-33.8135, -84.7252)
  line L56 (-33.8135, -84.7252) -> (-33.7586, -84.6686)
  arc A116 (-33.7586, -84.6686) -> (-33.8139, -77.6537) centre (-37.3495, -81.1892) ccw
  line L57 (-33.8139, -77.6537) -> (-38.5865, -72.8811)
  arc A117 (-38.9491, -66.2144) -> (-38.5865, -72.8811) centre (-35.0509, -69.3456) ccw
  arc A118 (-38.9441, -66.1678) -> (-38.9491, -66.2144) centre (-33.9744, -66.7173) ccw
  line L58 (-38.9441, -66.1678) -> (-36.0907, -63.3143)
  arc A119 (-32.277, -61.8576) -> (-36.0907, -63.3143) centre (-32.5552, -66.8499) ccw
  arc A120 (-32.277, -61.8576) -> (-29.6417, -59.2224) centre (-32.1379, -59.3615) ccw
  arc A121 (-28.185, -55.4086) -> (-29.6417, -59.2224) centre (-24.6495, -58.9442) ccw
  line L59 (-28.185, -55.4086) -> (-15.8059, -43.0296)
  arc A122 (-10.9963, -41.7301) -> (-15.8059, -43.0296) centre (-12.2704, -46.5651) ccw
  arc A123 (-10.9963, -41.7301) -> (10.9963, -41.7301) centre (0, 0) ccw
  arc A124 (15.8059, -43.0296) -> (10.9963, -41.7301) centre (12.2704, -46.5651) ccw
  line L60 (15.8059, -43.0296) -> (28.185, -55.4086)
  arc A125 (29.6417, -59.2224) -> (28.185, -55.4086) centre (24.6495, -58.9442) ccw
  arc A126 (-62.6322, -42.4797) -> (-62.2927, -49.1749) centre (-58.7571, -45.6394) ccw
  line L61 (-62.6322, -42.4797) -> (-43.4926, -23.3401)
  arc A127 (-35.8083, -24.0851) -> (-43.4926, -23.3401) centre (-39.9571, -26.8756) ccw
  arc A128 (-35.8083, -24.0851) -> (-24.0851, -35.8083) centre (0, 0) ccw
  arc A129 (-23.3401, -43.4926) -> (-24.0851, -35.8083) centre (-26.8756, -39.9571) ccw
  line L62 (-23.3401, -43.4926) -> (-42.122, -62.2745)
  arc A130 (-49.1931, -62.2745) -> (-42.122, -62.2745) centre (-45.6575, -58.739) ccw
  line L63 (-49.1931, -62.2745) -> (-62.2927, -49.1749)
  circle A131 centre (-32.1379, -59.3615) radius 1.75
  circle A132 centre (32.1379, -59.3615) radius 1.75
  circle A133 centre (69.3456, -45.6575) radius 1.75
  circle A134 centre (-45.6801, 69.3307) radius 1.75
  circle A135 centre (42.4052, 93.3169) radius 1.75
  circle A136 centre (45.6575, 69.3456) radius 1.75
  circle A137 centre (-93.3169, -42.4052) radius 1.75
  line L64 (72.863, -38.6046) -> (62.2927, -49.1749)
  circle A138 centre (-69.3307, -45.6801) radius 1.75
  circle A139 centre (69.3307, 45.6801) radius 1.75
  circle A140 centre (-93.3169, 42.4052) radius 1.75
  line L65 (38.6283, -72.8504) -> (49.1952, -62.2767)
  circle A141 centre (-69.3456, 45.6575) radius 1.75
  circle A142 centre (45.6801, -69.3307) radius 1.75
  circle A143 centre (-42.4052, -93.3169) radius 1.75
  circle A144 centre (-42.4052, 93.3169) radius 2.5
  line L66 (67.5778, -43.8898) -> (71.1134, -47.4253)
  line L67 (43.9118, -67.5635) -> (47.4484, -71.0979)
  circle A145 centre (-45.6575, -69.3456) radius 1.75
  circle A146 centre (42.4052, 93.3169) radius 2.5
  circle A147 centre (-42.4052, 93.3169) radius 1.75
  circle A148 centre (42.4052, -93.3169) radius 1.75
  circle A149 centre (93.3169, -42.4052) radius 1.75
  circle A150 centre (93.3169, 42.4052) radius 1.75
  point P0 (35.0916, -69.316)
  point P1 (38.2501, -65.4399)
  point P2 (41.7844, -61.9032)
  dimension "d99" = 3.5
  dimension "d100" = 3.5
  dimension "d101" = 3.5
  dimension "d102" = 3.5
  dimension "d103" = 3.5
  dimension "d104" = 3.5
  dimension "d105" = 3.5
  dimension "d106" = 3.5
  dimension "d107" = 5
  dimension "d108" = 5
  dimension "d109" = 3.5
  constraint coincident L66.start L64
  constraint midpoint A133.centre L66
  measures "d99" diameter of A149
  measures "d100" diameter of A150
  measures "d101" diameter of A148
  measures "d102" diameter of A143
  measures "d103" diameter of A137
  measures "d104" diameter of A140
  measures "d105" diameter of A135
  measures "d106" diameter of A147
  measures "d107" diameter of A146
  measures "d108" diameter of A144
  measures "d109" diameter of A133
extrude "押し出し14" cut sketch "スケッチ5" against normal blind 10 contours A5 A147 | A5 A147 | A28 A135 | A133 L66 | A133 L66 | A134 | A136 | A137 | A138 | A139 | A140 | A141 | A142 L67 | A142 L67 | A143 | A145 | A148 | A149 | A150 picked at (43.0238, 93.5186) bodies 1
extrude "押し出し15" add sketch "スケッチ5" against normal blind 1.5 contours A5 A144 A147 | A5 A144 A147 | A28 A135 A146 | A28 A135 A146 bodies 1
fillet "フィレット5" radius 2 4 edges at (40.6045, -91.5828, 0.75) (40.0961, -94.275, 0.75) (-40.6045, -91.5828, 0.75) (-40.0961, -94.275, 0.75) on bodies 1